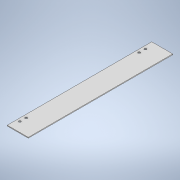
# Autodesk Inventor part: holder_wedge
Saved by Autodesk Inventor 2022 (Build 260153000, 153)
## iProperties
Created: 2021-11-26
Part Number: holder_wedge
Material: Generic
Document SubType Name: Modeling
Designer: Alex
Density: 1 g/cm^3
Appearance: Default
Author: Alex
Autodesk Inventor part; units mm, degrees
ref_plane "YZ Plane" through (0, 0, 0) normal (1, 0, 0) x (0, 1, 0)
ref_plane "XZ Plane" through (0, 0, 0) normal (0, 1, 0) x (-1, 0, 0)
ref_plane "XY Plane" through (0, 0, 0) normal (0, 0, 1) x (1, 0, 0)
sketch "Sketch1" plane through (0, 0, 0) normal (0, 1, 0) x (-1, 0, 0)
  line L0 (0, 0) -> (-42.418, 0)
  line L1 (-42.418, 0) -> (-42.418, -292.1)
  line L2 (-42.418, -292.1) -> (0, -292.1)
  line L3 (0, -292.1) -> (0, 0)
  circle A0 centre (-6.35, -19.05) radius 2.2225
  circle A1 centre (-6.35, -31.75) radius 2.2225
  circle A2 centre (-6.35, -273.05) radius 2.2225
  circle A3 centre (-6.35, -260.35) radius 2.2225
  dimension "d0" = 42.418
  dimension "d1" = 292.1
  dimension "d2" = 4.445
  dimension "d3" = 4.445
  dimension "d4" = 4.445
  dimension "d5" = 4.445
  constraints: 8 end point, 4 centre point, 2 parallel, 1 horizontal, 1 perpendicular
  measures "d0" distance of L2.end L1.end
  measures "d1" distance of L1.end L0.end
  measures "d2" diameter of A0
  measures "d3" diameter of A1
  measures "d4" diameter of A2
  measures "d5" diameter of A3
extrude "Extrusion1" add sketch "Sketch1" along normal blind 1.6002
body "Solid1"
